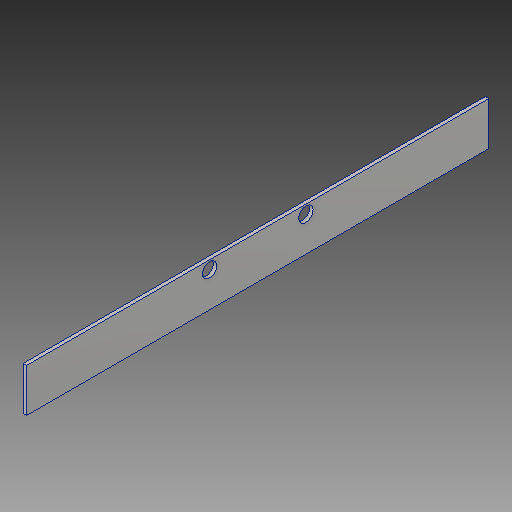
# Autodesk Inventor part: Inner Plate
Saved by Autodesk Inventor 2019.4 (Build 234330000, 330)
## iProperties
Created: 2019-12-07
Part Number: Inner Plate
Material: Aluminum 6061
Document SubType Name: Modeling
Designer: admin
Density: 2.7 g/cm^3
Appearance: Aluminum - Flat
Author: admin
Autodesk Inventor part; units mm, degrees
ref_plane "YZ Plane" through (0, 0, 0) normal (1, 0, 0) x (0, 1, 0)
ref_plane "XZ Plane" through (0, 0, 0) normal (0, 1, 0) x (-1, 0, 0)
ref_plane "XY Plane" through (0, 0, 0) normal (0, 0, 1) x (1, 0, 0)
sketch "Sketch1" plane through (0, 0, 0) normal (1, 0, 0) x (0, 1, 0)
  line L0 (49.2406, -510.0489) -> (-25.7594, -510.0489)
  line L1 (-25.7594, -510.0489) -> (-25.7594, 289.9511)
  line L2 (-25.7594, 289.9511) -> (49.2406, 289.9511)
  line L3 (49.2406, 289.9511) -> (49.2406, -510.0489)
  circle A0 centre (34.2406, -193.3994) radius 12.5
  circle A1 centre (34.2406, -26.6984) radius 12.5
  line L4 (34.2406, -193.3994) -> (34.2406, -26.6984) construction
  line L5 (34.2406, -110.0489) -> (2.7957, -110.0489) construction
  point P0 (0, 0)
  dimension "d2" = 75
  dimension "d3" = 800
  dimension "d4" = 25
  dimension "d5" = 25
  dimension "d7" = 166.701
  dimension "d8" = 60
  dimension "d9" = 400
  constraints: 12 end point, 2 centre point, 2 horizontal, 2 parallel, 1 midpoint, 1 perpendicular, 1 vertical
  measures "d2" distance of L0.start L0.end
  measures "d3" distance of L2.end L0.start
  measures "d4" diameter of A0
  measures "d5" diameter of A1
  measures "d7" distance of L4.end L4.start
  measures "d8" distance between parallel lines of L1 L4
  measures "d9" distance between parallel lines of L0 L5
extrude "Extrusion1" add sketch "Sketch1" along normal blind 6
equation "\"d9\" = 0.5 * d3"
body "Solid1"
